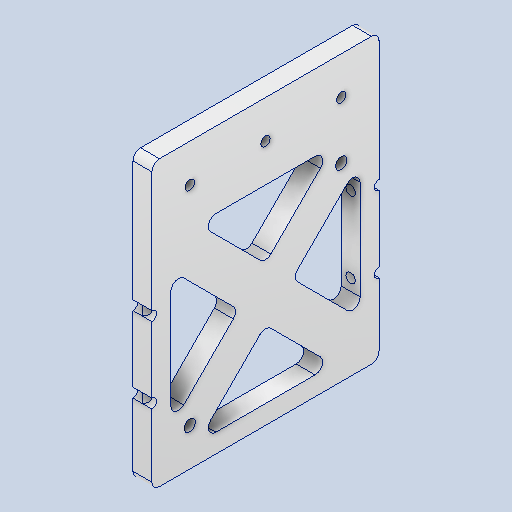
# Autodesk Inventor part: base_weel-v3-Plate-8
Saved by Autodesk Inventor 2025.2 (Build 292293000, 293)
## iProperties
Created: 2025-04-05
Part Number: base_weel-v3-Plate-8
Material: アルミニウム 6061
Document SubType Name: Modeling
Designer: haruy
Density: 2.7 g/cm^3
Appearance: アルミニウム - フラット
Author: haruy
Autodesk Inventor part; units mm, degrees
ref_plane "YZ Plane" through (0, 0, 0) normal (1, 0, 0) x (0, 1, 0)
ref_plane "XZ Plane" through (0, 0, 0) normal (0, 1, 0) x (-1, 0, 0)
derived "base_weel-v3-ASP-Base.ipt"
sketch "スケッチ9" plane through (0, -300, -190) normal (1, 0, 0) x (0, 0, -1)
  line L0 (-215, 0) -> (-165, 0) projected
  line L1 (-165, 0) -> (-165, -50) projected
  line L2 (-165, -50) -> (-215, -50) projected
  line L3 (-215, -50) -> (-215, 0) projected
  circle A0 centre (-190, -25) radius 22 projected
  line L4 (-212, -25) -> (-168, -25) projected
  line L5 (-380, 0) -> (0, 0) projected
  line L6 (-268.5, 20) -> (-268.5, 241.5) projected
  line L7 (-220, 20) -> (-160, 20) projected
  line L8 (-160, 20) -> (-160, -55) projected
  line L9 (-160, -55) -> (-220, -55) projected
  line L10 (-220, -55) -> (-220, 20) projected
  circle A1 centre (-170, -5) radius 1.5 projected
  line L11 (0, 20) -> (-380, 20) projected
  circle A2 centre (-210, 10) radius 1.25 projected
  circle A3 centre (-190, 10) radius 1.25 projected
  circle A4 centre (-210, -45) radius 1.5
  circle A5 centre (-190, 300) radius 360 projected
  circle A6 centre (-210, -45) radius 1.6 projected
  circle A7 centre (-170, 10) radius 1.25 projected
  circle A8 centre (-190, -25) radius 10
  line L12 (-215, -50) -> (-190, -25)
  line L13 (-218.5355, -46.4645) -> (-193.5355, -21.4645)
  line L14 (-211.4645, -53.5355) -> (-186.4645, -28.5355)
  line L15 (-190, -25) -> (-190, -50)
  line L16 (-161.4645, -46.4645) -> (-186.4645, -21.4645)
  line L17 (-168.5355, -53.5355) -> (-193.5355, -28.5355)
  line L18 (-218.5355, -3.5355) -> (-193.5355, -28.5355)
  line L19 (-211.4645, 3.5355) -> (-186.4645, -21.4645)
  line L20 (-168.5355, 3.5355) -> (-193.5355, -21.4645)
  line L21 (-161.4645, -3.5355) -> (-186.4645, -28.5355)
  point P0 (-215, -42.9289)
  point P1 (-215, -7.0711)
  point P2 (-197.0711, -25)
  point P3 (-182.9289, -25)
  point P4 (-165, -7.0711)
  point P5 (-165, -42.9289)
  point P6 (-207.9289, 0)
  point P7 (-172.0711, 0)
  point P8 (-190, -17.9289)
  point P9 (-190, -32.0711)
  point P10 (-172.0711, -50)
  point P11 (-207.9289, -50)
  dimension "d1" = 3
  dimension "d2" = 5
  dimension "d3" = 5
  dimension "d6" = 20
  dimension "d7" = 5
  dimension "d8" = 5
  constraints: 20 end point, 12 symmetric about line, 2 centre point, 2 parallel, 1 coincident, 1 midpoint, 1 perpendicular
  measures "d1" diameter of A4
  measures "d2" distance from line of A4.centre L2
  measures "d3" distance from line of A4.centre L3
  measures "d6" diameter of A8
  measures "d7" distance between parallel lines of L12 L13
  measures "d8" distance between parallel lines of L12 L14
extrude "押し出し1" add sketch "スケッチ9" against normal blind 5 contours L5 L10 L7 L8 L0 | L0 L19 A0 L18 L3 | L3 L2 L1 L5 L8 L9 L10 | L0 L1 L21 A0 L20 | L19 A8 L18 A0 | L13 A0 L12 A6 L3 | A0 L21 A8 L20 | L19 L20 L13 L18 A8 | L12 A6 A0 L14 L2 | L13 A8 L12 A0 | A8 L21 L16 L19 L20 | L19 L16 L4 L13 L20 | L12 A4 A6 | A6 L12 A4 | L12 A8 L14 A0 | L13 L18 L12 A8 | L4 L12 L18 | L1 L2 L17 A0 L16 | L12 L17 L14 A8 | L15 L17 L12 | L4 L21 L14 L15 | A0 L17 A8 L16 | L16 A8 L17 L14 L21
fillet "フィレット1" radius 2 12 edges at (-2.5, -332.0711, 0) (-2.5, -350, 17.9289) (-2.5, -350, -17.9289) (-2.5, -342.9289, -25) (-2.5, -325, -7.0711) (-2.5, -307.0711, -25) (-2.5, -307.0711, 25) (-2.5, -325, 7.0711) (-2.5, -342.9289, 25) (-2.5, -317.9289, 0) (-2.5, -300, 17.9289) (-2.5, -300, -17.9289)
sketch "スケッチ2" plane through (0, -355, 30) normal (0, 0, 1) x (1, 0, 0)
  line L0 (-5, 55) -> (-40, 55)
  line L1 (-40, 55) -> (-40, 5)
  line L2 (-40, 5) -> (-5, 5)
  line L3 (-5, 5) -> (-5, 55)
  line L4 (-40, 52) -> (-75, 52)
  line L5 (-75, 52) -> (-75, 8)
  line L6 (-75, 8) -> (-40, 8)
  line L7 (-40, 8) -> (-40, 52)
  line L8 (0, 0) -> (-5, 0) projected
  line L9 (-5, 0) -> (-5, 75) projected
  line L10 (0, 75) -> (-5, 75) projected
  line L11 (0, 75) -> (20, 75)
  line L12 (20, 75) -> (20, 55)
  line L13 (20, 55) -> (0, 55)
  line L14 (0, 55) -> (0, 75)
  line L15 (-75, 60) -> (-70, 60)
  line L16 (-70, 60) -> (-70, 0)
  line L17 (-70, 0) -> (-75, 0)
  line L18 (-75, 0) -> (-75, 60)
  line L19 (-5, 75) -> (-75, 75)
  line L20 (-75, 75) -> (-75, 55)
  line L21 (-75, 55) -> (-5, 55)
  line L22 (-5, 55) -> (-5, 75)
  line L23 (-5, 0) -> (-40, 55)
  line L24 (0, 75) -> (-5, 75)
  line L25 (-5, 75) -> (-5, 0)
  line L26 (-5, 0) -> (0, 0)
  line L27 (0, 0) -> (0, 75)
  line L28 (0, 37.5) -> (-5, 37.5)
  line L29 (-37.5, 75) -> (-37.5, 0)
  circle A0 centre (-2.5, 30) radius 1.5
  circle A1 centre (-2.5, 40) radius 1.5
  circle A2 centre (-2.5, 20) radius 1.5
  circle A3 centre (-72.5, 30) radius 1.5
  circle A4 centre (-72.5, 40) radius 1.5
  circle A5 centre (-72.5, 20) radius 1.5
  point P0 (0, 355)
  dimension "d10" = 35
  dimension "d11" = 50
  dimension "d12" = 35
  dimension "d13" = 44
  dimension "d14" = 3
  dimension "d15" = 5
  dimension "d16" = 0
  dimension "d17" = 20
  dimension "d18" = 20
  dimension "d19" = 5
  dimension "d20" = 0
  dimension "d21" = 0
  dimension "d22" = 5
  dimension "d23" = 0
  dimension "d24" = 0
  dimension "d26" = 37.5
  dimension "d27" = 3
  dimension "d28" = 25
  dimension "d29" = 2.5
  dimension "d30" = 3
  dimension "d31" = 3
  dimension "d32" = 2.5
  dimension "d33" = 2.5
  dimension "d34" = 10
  dimension "d35" = 10
  constraints: 54 end point, 12 parallel, 6 centre point, 6 horizontal, 6 perpendicular, 3 symmetric about line, 2 midpoint, 2 point on line, 1 vertical, 3 other
  measures "d10" distance of L2.end L1.end
  measures "d11" distance of L1.end L0.end
  measures "d12" distance of L6.end L5.end
  measures "d13" distance of L5.end L4.end
  measures "d14" distance between parallel lines of L0 L4
  measures "d15" distance between parallel lines of L8 L2
  measures "d16" distance between parallel lines of L3 L9
  measures "d17" distance of L12.end L13.end
  measures "d18" distance of L11.end L12.end
  measures "d19" distance of L16.end L17.end
  measures "d20" distance between parallel lines of L5 L18
  measures "d21" distance between parallel lines of L17 L8
  measures "d22" distance between parallel lines of L15 L0
  measures "d23" distance between parallel lines of L21 L0
  measures "d24" distance between parallel lines of L18 L20
  measures "d26" distance between parallel lines of L29 L14
  measures "d27" diameter of A0
  measures "d28" distance from line of A0.centre L21
  measures "d29" distance from line of A0.centre L3
  measures "d30" diameter of A1
  measures "d31" diameter of A2
  measures "d32" distance from line of A1.centre L3
  measures "d33" distance from line of A2.centre L3
  measures "d34" distance of A1.centre A0.centre
  measures "d35" distance of A2.centre A0.centre
hole "穴1" at (-2.5, -315, 30) at (-2.5, -335, 30) direction (0, 0, -1) diameter 2.5 depth 5 tip angle 118
fillet "フィレット2" radius 2 4 edges at (-2.5, -355, 30) (-2.5, -355, -30) (-2.5, -280, 30) (-2.5, -280, -30)
ref_plane "作業平面1" through (0, -353, 0) normal (0, 0, 1) x (1, 0, 0)
mirror "ミラー1" about plane through (0, -353, 0) normal (0, 0, 1) of "穴1"
sketch "スケッチ3" plane through (0, -353, 30) normal (1, 0, 0) x (0, 0, -1)
  line L0 (0, 0) -> (0, 71) projected
  circle A0 centre (0, 38) radius 1.25
  line L1 (2, -2) -> (58, -2) projected
  circle A1 centre (0, 18) radius 1.25
  line L2 (2, 73) -> (58, 73) projected
  line L3 (30, 73) -> (30, -2)
  circle A2 centre (60, 38) radius 1.25
  circle A3 centre (60, 18) radius 1.25
  point P0 (30, 353)
  dimension "d45" = 2.5
  dimension "d46" = 40
  dimension "d47" = 2.5
  dimension "d48" = 20
  constraints: 4 centre point, 2 end point, 2 midpoint, 2 point on line, 2 symmetric about line, 2 other
  measures "d45" diameter of A0
  measures "d46" distance from line of A0.centre L1
  measures "d47" diameter of A1
  measures "d48" distance of A1.centre A0.centre
extrude "押し出し2" cut sketch "スケッチ3" against normal blind 10
equation "\"d8\" = d7"
equation "\"d32\" = d29"
equation "\"d33\" = d29"
equation "\"d35\" = d34"
